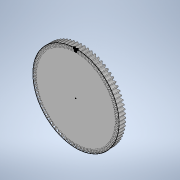
# Autodesk Inventor part: dial_gear
Saved by Autodesk Inventor 2021 (Build 250183000, 183)
## iProperties
Created: 2021-05-06
Part Number: dial_gear
Material: Generic
Document SubType Name: Modeling
Designer: froppy
Density: 1 g/cm^3
Appearance: Default
Author: froppy
Autodesk Inventor part; units mm, degrees
ref_plane "YZ Plane" through (0, 0, 0) normal (1, 0, 0) x (0, 1, 0)
ref_plane "XZ Plane" through (0, 0, 0) normal (0, 1, 0) x (-1, 0, 0)
ref_plane "XY Plane" through (0, 0, 0) normal (0, 0, 1) x (1, 0, 0)
sketch "Sketch1" plane through (0, 0, 0) normal (0, 0, 1) x (1, 0, 0)
  spline S0 degree 3 poles (-1.2975, 38.4781) (-1.2456, 38.3683) (-1.1416, 38.1487) (-0.9963, 37.8144) (-0.8592, 37.4767) (-0.732, 37.1351) (-0.615, 36.7899) (-0.5375, 36.5277) (-0.4879, 36.3524) (-0.4529, 36.2679) (-0.4124, 36.2034) (-0.3742, 36.156) (-0.3403, 36.1255) (-0.3054, 36.096) (-0.2658, 36.0733) (-0.2249, 36.053) (-0.1812, 36.0399) (-0.1367, 36.0296) (-0.0759, 36.026) (0, 36.028) (0.0759, 36.026) (0.1367, 36.0296) (0.1812, 36.0399) (0.2249, 36.053) (0.2658, 36.0733) (0.3054, 36.096) (0.3403, 36.1255) (0.3742, 36.156) (0.4124, 36.2034) (0.4529, 36.2679) (0.4879, 36.3524) (0.5375, 36.5277) (0.615, 36.7899) (0.732, 37.1351) (0.8592, 37.4767) (0.9963, 37.8144) (1.1416, 38.1487) (1.2456, 38.3683) (1.2975, 38.4781) knots 0 0 0 0 0.036445 0.07289 0.109334 0.145779 0.182223 0.218667 0.227775 0.23688 0.24598 0.250536 0.25509 0.259642 0.264198 0.268751 0.273304 0.277859 0.282414 0.291525 0.300637 0.305192 0.309747 0.314299 0.318853 0.323408 0.327961 0.332514 0.337071 0.346171 0.355275 0.364384 0.400828 0.437272 0.473717 0.510161 0.546606 0.583051 0.583051 0.583051 0.583051
  circle A0 centre (0, 0) radius 36.0272 construction
  circle A1 centre (0, 0) radius 35.2385 construction
  circle A2 centre (0, 0) radius 37.5 construction
  circle A3 centre (0, 0) radius 38.5
  point P0 (-1.1434, 38.1479)
  point P1 (-0.9977, 37.8138)
  point P2 (-0.8608, 37.476)
  point P3 (-0.7337, 37.1345)
  point P4 (-0.6173, 36.7892)
  point P5 (-0.5128, 36.44)
  point P6 (-0.4862, 36.3529)
  point P7 (-0.4506, 36.2691)
  point P8 (-0.4024, 36.1919)
  point P9 (-0.3733, 36.1568)
  point P10 (-0.3402, 36.1256)
  point P11 (-0.3047, 36.0971)
  point P12 (-0.2656, 36.0737)
  point P13 (-0.2245, 36.0542)
  point P14 (-0.1811, 36.0404)
  point P15 (-0.1365, 36.0309)
  point P16 (-0.0911, 36.0273)
  point P17 (0, 36.0272)
  point P18 (0.0911, 36.0273)
  point P19 (0.1365, 36.0309)
  point P20 (0.1811, 36.0404)
  point P21 (0.2245, 36.0542)
  point P22 (0.2656, 36.0737)
  point P23 (0.3047, 36.0971)
  point P24 (0.3402, 36.1256)
  point P25 (0.3733, 36.1568)
  point P26 (0.4024, 36.1919)
  point P27 (0.4506, 36.2691)
  point P28 (0.4862, 36.3529)
  point P29 (0.5128, 36.44)
  point P30 (0.6173, 36.7892)
  point P31 (0.7337, 37.1345)
  point P32 (0.8608, 37.476)
  point P33 (0.9977, 37.8138)
  point P34 (1.1434, 38.1479)
  constraints: 4 centre point, 2 point on circle, 79 other
extrude "Extrusion1" add sketch "Sketch1" against normal blind 6.35
extrude "Extrusion2" cut sketch "Sketch1" against normal through all contours A3 S0 picked at (-0.0702, 37.4988)
pattern_circular "Circular Pattern1" count 75 over 360 about axis through (0, 0, -10) along (0, 0, 1) of "Extrusion2"
sketch "Sketch2" plane through (0, 0, -6.35) normal (0, 0, -1) x (-1, 0, 0)
  line L0 (2.3812, 2.1001) -> (-2.3813, 2.1001)
  line L1 (-2.3813, 2.1001) -> (-2.3812, -2.1001)
  line L2 (-2.3812, -2.1001) -> (2.3813, -2.1001)
  line L3 (2.3813, -2.1001) -> (2.3812, 2.1001)
  circle A0 centre (0, 0) radius 3.175
  circle A1 centre (0, 0) radius 3.9688
  point P0 (2.3813, -2.1001)
  dimension "d7" = 4.7625
  dimension "d8" = 6.35
  dimension "d9" = 0.7937
  constraints: 8 end point, 3 point on circle, 2 centre point, 2 coincident, 2 parallel, 1 horizontal, 1 perpendicular
  measures "d7" distance between parallel lines of L3 L1
  measures "d8" diameter of A0
  measures "d9" radial gap between concentric circles of A0 A1
extrude "Extrusion3" add sketch "Sketch2" along normal blind 19.05 contours A0 L3 | L1 A0 | A1
sketch "Sketch3" plane through (0, 0, -6.35) normal (0, 0, -1) x (-1, 0, 0)
  line L0 (2.3813, -2.1001) -> (2.3812, 2.1001) projected
  arc A0 (2.3812, 2.1001) -> (-2.3813, 2.1001) centre (0, 0) ccw projected
  line L1 (-2.3813, 2.1001) -> (-2.3812, -2.1001) projected
  arc A1 (-2.3812, -2.1001) -> (2.3813, -2.1001) centre (0, 0) ccw projected
extrude "Extrusion4" add sketch "Sketch3" along normal blind 12.7
equation "\"d0\" = FaceWidth"
equation "\"Module\" = 1"
equation "\"PressureAngle\" = 20deg"
equation "\"UnitProfileClearance\" = 0.25"
equation "\"UnitRoundRadius\" = 0.35"
equation "\"HeadDiameter\" = 77"
equation "\"RootDiameter\" = 72.05441"
equation "\"BaseDiameter\" = 70.47695"
equation "\"PitchDiameter\" = 75"
equation "\"FaceWidth\" = 6.35"
equation "\"HelixAngle\" = 0"
equation "\"UnitCorrection\" = 0"
equation "\"UnitAddendumModification\" = 0"
equation "\"CircularPitch\" = 3.141593"
equation "\"UnitBacklashShift\" = -0.222794"
equation "\"TotalToolShift\" = -0.22279"
equation "\"IsInternal\" = 0"
body "Solid1"
